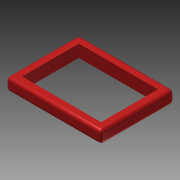
# Autodesk Inventor part: bumpers
Saved by Autodesk Inventor 2014 (Build 180170000, 170)
## iProperties
Created: 2014-01-07
Part Number: bumpers
Material: Generic
Document SubType Name: Modeling
Designer: pc
Density: 1 g/cm^3
Appearance: Light Red
Author: pc
Autodesk Inventor part; units mm, degrees
ref_plane "YZ Plane" through (0, 0, 0) normal (1, 0, 0) x (0, 1, 0)
ref_plane "XZ Plane" through (0, 0, 0) normal (0, 1, 0) x (-1, 0, 0)
ref_plane "XY Plane" through (0, 0, 0) normal (0, 0, 1) x (1, 0, 0)
sketch "Sketch1" plane through (0, 0, 0) normal (0, 1, 0) x (-1, 0, 0)
  line L0 (0, 0) -> (812.8, 0)
  line L1 (812.8, 0) -> (812.8, -584.2)
  line L2 (812.8, -584.2) -> (0, -584.2)
  line L3 (0, -584.2) -> (0, 0)
  line L4 (-82.55, 82.55) -> (895.35, 82.55)
  line L5 (895.35, 82.55) -> (895.35, -666.75)
  line L6 (895.35, -666.75) -> (-82.55, -666.75)
  line L7 (-82.55, -666.75) -> (-82.55, 82.55)
  dimension "d0" = 812.8
  dimension "d1" = 584.2
  dimension "d2" = 82.55
  dimension "d3" = 82.55
  dimension "d4" = 82.55
  dimension "d5" = 82.55
  constraints: 16 end point, 4 parallel, 2 horizontal, 2 perpendicular
  measures "d0" distance of L1.end L2.end
  measures "d1" distance of L0.end L1.end
  measures "d2" distance between parallel lines of L0 L4
  measures "d3" distance between parallel lines of L2 L6
  measures "d4" distance between parallel lines of L1 L5
  measures "d5" distance between parallel lines of L3 L7
extrude "Extrusion1" add sketch "Sketch1" along normal blind 127
fillet "Fillet1" radius 31.75 8 edges at (-406.4, 127, 82.55) (82.55, 127, -292.1) (-406.4, 0, 82.55) (82.55, 0, -292.1) (-895.35, 127, -292.1) (-406.4, 127, -666.75) (-406.4, 0, -666.75) (-895.35, 0, -292.1)
fillet "Fillet2" radius 31.75 12 edges at (-886.0506, 117.7006, 73.2506) (-886.0506, 9.2994, 73.2506) (-895.35, 63.5, 82.55) (-886.0506, 117.7006, -657.4506) (-886.0506, 9.2994, -657.4506) (-895.35, 63.5, -666.75) (73.2506, 117.7006, 73.2506) (73.2506, 9.2994, 73.2506) (82.55, 63.5, 82.55) (73.2506, 117.7006, -657.4506) (73.2506, 9.2994, -657.4506) (82.55, 63.5, -666.75)
body "Solid1"
